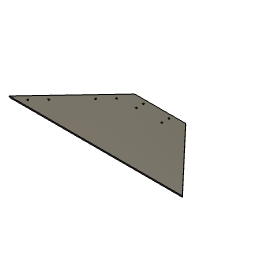
Right (Autodesk Fusion 360 design; units mm, degrees)
Autodesk Fusion 360 part; units mm, degrees
sketch "Sketch1" plane through (0, 0, 0) normal (0, 1, 0) x (1, 0, 0)
  line L0 (0, 0) -> (431.8, 0)
  line L1 (215.9, 160.6296) -> (152.4, 160.6296)
  line L2 (215.9, 160.6296) -> (279.4, 160.6296)
  line L3 (279.4, 160.6296) -> (431.8, 0)
  line L4 (152.4, 160.6296) -> (0, 0)
  circle A0 centre (247.65, 132.6896) radius 1.905
  circle A1 centre (113.9739, 101.6767) radius 1.905
  circle A2 centre (31.5031, 14.7524) radius 1.905
  circle A3 centre (139.3232, 128.3949) radius 1.905
  circle A4 centre (184.15, 150.4696) radius 1.905
  circle A5 centre (56.8524, 41.4706) radius 1.905
  circle A6 centre (247.65, 150.4696) radius 1.905
  circle A7 centre (184.15, 132.6896) radius 1.905
  dimension "d1" = 431.8
  dimension "d3" = 63.5
  dimension "d4" = 63.5
  constraint coincident L0.start L4.end
  constraint horizontal L0
  measures "d1" distance of L0.start L0.end
  measures "d3" distance of L1.start L1.end
  measures "d4" distance of L1.start L2.end
extrude "Extrude5" add sketch "Sketch1" along normal blind 2.794
